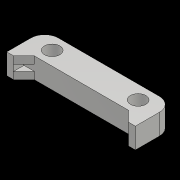
# Autodesk Inventor part: dcdcfixer
Saved by Autodesk Inventor 2018.2 (Build 222227000, 227)
## iProperties
Created: 2019-11-16
Part Number: dcdcfixer
Material: アルミニウム 6061
Document SubType Name: Modeling
Designer: gisen
Density: 2.7 g/cm^3
Appearance: アルミニウム - フラット
Author: gisen
## iProperties of the stored document dcdcfixer_3D プリント.ipt
Created: 2019-11-17
Part Number: dcdcfixer_3D プリント
Material: アルミニウム 6061
Document SubType Name: Modeling
Designer: gisen
Density: 2.7 g/cm^3
Appearance: アルミニウム - フラット
Author: gisen
Autodesk Inventor part; units mm, degrees
ref_plane "YZ Plane" through (0, 0, 0) normal (1, 0, 0) x (0, 1, 0)
ref_plane "XZ Plane" through (0, 0, 0) normal (0, 1, 0) x (-1, 0, 0)
ref_plane "XY Plane" through (0, 0, 0) normal (0, 0, 1) x (1, 0, 0)
sketch "スケッチ1" plane through (0, 0, 0) normal (0, 0, 1) x (1, 0, 0)
  line L0 (-16.7, 1.5) -> (16.7, 1.5) construction
  line L1 (16.7, 1.5) -> (16.7, -1.5) construction
  line L2 (16.7, -1.5) -> (-16.7, -1.5) construction
  line L3 (-16.7, -1.5) -> (-16.7, 1.5) construction
  line L4 (-16.7, 1.5) -> (16.7, -1.5) construction
  line L5 (16.7, 1.5) -> (-16.7, -1.5) construction
  line L6 (-16.7, -1.5) -> (-16.7, 1.5)
  line L7 (-16.7, 1.5) -> (16.7, 1.5)
  line L8 (16.7, 1.5) -> (16.7, -1.5)
  line L9 (16.7, -1.5) -> (18.7, -1.5)
  line L10 (18.7, -1.5) -> (18.7, 9.5)
  line L11 (18.7, 9.5) -> (-18.7, 9.5)
  line L12 (-18.7, 9.5) -> (-18.7, -1.5)
  line L13 (-18.7, -1.5) -> (-16.7, -1.5)
  circle A0 centre (-12.5, 5.5) radius 2.25
  line L14 (0, 9.5) -> (0, 0) construction
  circle A1 centre (12.5, 5.5) radius 2.25
  dimension "d0" = 3
  dimension "d1" = 33.4
  dimension "d2" = 8
  dimension "d3" = 2
  dimension "d4" = 4.5
  dimension "d5" = 4
  dimension "d6" = 6.2
  constraints: 30 end point, 8 perpendicular, 3 midpoint, 2 centre point, 2 parallel, 2 vertical, 1 collinear, 1 horizontal, 1 point on line, 1 symmetric about line, 1 other
  measures "d0" distance of L0.end L1.end
  measures "d1" distance of L0.start L0.end
  measures "d2" distance between parallel lines of L7 L11
  measures "d3" distance of L12.end L2.end
  measures "d4" diameter of A0
  measures "d5" distance from line of A0.centre L11
  measures "d6" distance from line of L12 A0.centre
extrude "押し出し1" add sketch "スケッチ1" along normal blind 1.8
sketch "スケッチ2" plane through (0, 0, 1.8) normal (0, 0, 1) x (1, 0, 0)
  line L0 (-18.7, -1.5) -> (-16.7, -1.5)
  line L1 (-16.7, -1.5) -> (-13.7, 1.5)
  line L2 (-13.7, 1.5) -> (13.7, 1.5)
  line L3 (13.7, 1.5) -> (16.7, -1.5)
  line L4 (16.7, -1.5) -> (18.7, -1.5)
  line L5 (18.7, -1.5) -> (18.7, 9.5)
  line L6 (18.7, 9.5) -> (-18.7, 9.5)
  line L7 (-18.7, 9.5) -> (-18.7, -1.5)
  line L8 (-16.7, 1.5) -> (16.7, 1.5) projected
  circle A0 centre (-12.5, 5.5) radius 2.25 projected
  circle A1 centre (12.5, 5.5) radius 2.25 projected
  point P0 (0, 0)
  dimension "d9" = 135
  dimension "d10" = 135
  constraints: 16 end point, 3 perpendicular, 2 coincident, 1 collinear, 1 horizontal, 1 parallel, 1 point on line
  measures "d9" angle of L0 L1
  measures "d10" angle of L4 L3
extrude "押し出し2" add sketch "スケッチ2" along normal blind 2.1
sketch "スケッチ3" plane through (0, 0, 0) normal (0, 0, -1) x (-1, 0, 0)
  circle A0 centre (-12.5, 5.5) radius 2.25 projected
  circle A1 centre (12.5, 5.5) radius 2.25 projected
  line L0 (18.7, -1.5) -> (16.7, -1.5) projected
  line L1 (16.7, -1.5) -> (13.7, 1.5) projected
  line L2 (13.7, 1.5) -> (-13.7, 1.5) projected
  line L3 (-13.7, 1.5) -> (-16.7, -1.5) projected
  line L4 (-16.7, -1.5) -> (-18.7, -1.5) projected
  line L5 (-18.7, -1.5) -> (-18.7, 9.5) projected
  line L6 (-18.7, 9.5) -> (18.7, 9.5) projected
  line L7 (18.7, 9.5) -> (18.7, -1.5) projected
  point P0 (0, 0)
extrude "押し出し3" add sketch "スケッチ3" along normal blind 2.1
fillet "フィレット1" radius 4 2 edges at (18.7, 9.5, 0.9) (-18.7, 9.5, 0.9)
equation "\"d5\" = 0.5 * d2"
equation "\"d10\" = d9"
